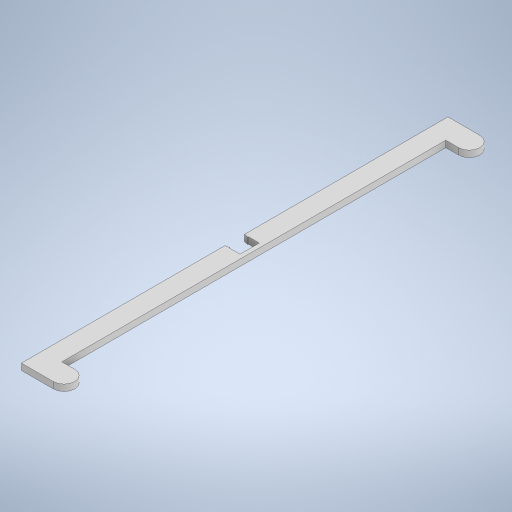
# Autodesk Inventor part: Lower_Bar_3
Saved by Autodesk Inventor 2024 (Build 280153000, 153)
## iProperties
Created: 2024-04-09
Part Number: Lower_Bar_3
Material: 一般
Document SubType Name: Modeling
Designer: USER
Density: 1 g/cm^3
Appearance: 預設
Author: USER
Autodesk Inventor part; units mm, degrees
ref_plane "YZ Plane" through (0, 0, 0) normal (1, 0, 0) x (0, 1, 0)
ref_plane "XZ Plane" through (0, 0, 0) normal (0, 1, 0) x (-1, 0, 0)
ref_plane "XY Plane" through (0, 0, 0) normal (0, 0, 1) x (1, 0, 0)
sketch "草圖1" plane through (0, 0, 0) normal (0, 1, 0) x (-1, 0, 0)
  line L0 (0, 90) -> (9, 90)
  line L1 (9, -90) -> (0, -90)
  line L2 (0, -90) -> (0, 90)
  line L3 (7, 4.5) -> (2, 4.5)
  line L4 (2, 4.5) -> (2, -4.5)
  line L5 (2, -4.5) -> (7, -4.5)
  line L6 (9, 90) -> (9, 100)
  line L7 (9, 100) -> (-6, 100)
  line L8 (-11, 95) -> (-11, 95)
  line L9 (-6, 90) -> (0, 90)
  arc A0 (-11, 95) -> (-6, 90) centre (-6, 95) ccw
  arc A1 (-6, 100) -> (-11, 95) centre (-6, 95) ccw
  circle A2 centre (-6, 95) radius 2.5
  line L10 (9, 0) -> (0, 0)
  line L11 (9, -90) -> (9, -100)
  line L12 (9, -100) -> (-6, -100)
  line L13 (-6, -90) -> (0, -90)
  arc A3 (-6, -90) -> (-11, -95) centre (-6, -95) ccw
  arc A4 (-11, -95) -> (-6, -100) centre (-6, -95) ccw
  circle A5 centre (-6, -95) radius 2.5
  line L14 (9, 90) -> (9, 4.6)
  line L15 (9, -4.6) -> (9, -90)
  line L16 (7, -4.5) -> (7, -4.2)
  line L17 (7, -4.2) -> (9, -4.6)
  line L18 (7, 4.5) -> (7, 4.2)
  line L19 (7, 4.2) -> (9, 4.6)
  point P0 (4.5, 4.5)
  point P1 (4.5, 90)
  point P2 (-11, 100)
  point P3 (-11, -100)
  point P4 (2, 0)
  dimension "d0" = 180
  dimension "d1" = 9
  dimension "d3" = 5
  dimension "d4" = 10
  dimension "d5" = 20
  dimension "d6" = 5
  dimension "d7" = 5
  dimension "d8" = 5
  dimension "d11" = 85.4
  dimension "d12" = 85.4
  dimension "d13" = 9
  dimension "d14" = 0.3
  dimension "d15" = 0.3
  dimension "d16" = 11.31
  dimension "d17" = 0
  dimension "d18" = 5
  dimension "d19" = 20
  dimension "d20" = 185
  dimension "d21" = 20
  constraints: 40 end point, 9 symmetric about line, 8 point on circle, 6 centre point, 6 perpendicular, 5 parallel, 4 midpoint, 4 tangent, 3 coincident, 3 horizontal, 3 point on line, 3 vertical, 1 horizontal alignment, 1 vertical alignment, 3 other
  measures "d0" distance of L0.end L1.start
  measures "d1" distance of L0.start L0.end
  measures "d3" distance of L4.end L5.end
  measures "d4" distance of L0.end L6.end
  measures "d5" distance of L6.end point (-11, 100)
  measures "d6" radius of A0
  measures "d7" radius of A1
  measures "d8" diameter of A2
  measures "d11" distance of L0.end L14.end
  measures "d12" distance of L15.start L1.start
  measures "d13" distance of L3.end L4.end
  measures "d14" distance of L5.end L16.end
  measures "d15" distance of L3.start L18.end
  measures "d16" angle of L0 L19
  measures "d17" distance from line of L10.start L15
  measures "d18" distance from line of point (-11, 95) L0
  measures "d19" distance from line of point (-11, 95) L15
  measures "d20" distance from line of point (-11, -95) L0
  measures "d21" distance from line of point (-11, -95) L15
extrude "擠出1" add sketch "草圖1" along normal blind 3 contours L9 A0 A1 L7 L6 L0 | L0 L14 L19 L18 L3 L4 L10 L2 | L10 L4 L5 L16 L17 L15 L1 L2 | L1 L11 L12 A4 A3 L13 | A2 | A5
